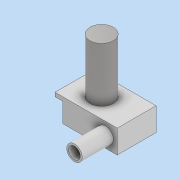
# Autodesk Inventor part: TuningPeg
Saved by Autodesk Inventor 2021 (Build 250183000, 183)
## iProperties
Created: 2021-02-02
Part Number: TuningPeg
Material: Generic
Document SubType Name: Modeling
Designer: garre
Density: 1 g/cm^3
Appearance: Default
Author: garre
Autodesk Inventor part; units mm, degrees
ref_plane "YZ Plane" through (0, 0, 0) normal (1, 0, 0) x (0, 1, 0)
ref_plane "XZ Plane" through (0, 0, 0) normal (0, 1, 0) x (-1, 0, 0)
ref_plane "XY Plane" through (0, 0, 0) normal (0, 0, 1) x (1, 0, 0)
sketch "Sketch1" plane through (0, 0, 0) normal (0, 1, 0) x (-1, 0, 0)
  circle A0 centre (0, 0) radius 4.7625
  line L0 (0, 0) -> (-14.2875, 0)
  line L1 (-14.2875, 0) -> (-14.2875, 7.9375)
  line L2 (-14.2875, 7.9375) -> (7.9375, 7.9375)
  line L3 (7.9375, 7.9375) -> (7.9375, -7.9375)
  line L4 (7.9375, -7.9375) -> (-14.2875, -7.9375)
  line L5 (-14.2875, -7.9375) -> (-14.2875, 7.9375)
  line L6 (0, -7.9375) -> (11.1125, -7.9375)
  line L7 (11.1125, -7.9375) -> (11.1125, 7.9375)
  line L8 (11.1125, 7.9375) -> (0, 7.9375)
  line L9 (0, 7.9375) -> (0, -7.9375)
  dimension "d0" = 9.525
  dimension "d9" = 15.875
  dimension "d10" = 7.9375
  dimension "d11" = 14.2875
  dimension "d12" = 7.9375
  dimension "d22" = 11.1125
  constraints: 20 end point, 4 parallel, 3 horizontal, 2 perpendicular, 1 centre point, 1 coincident, 1 midpoint, 1 point on line, 1 vertical
  measures "d0" diameter of A0
  measures "d9" distance of L4.end L1.end
  measures "d10" distance of L0.end L1.end
  measures "d11" distance from line of L5 point (0, 0)
  measures "d12" distance from line of L3 point (0, 0)
  measures "d22" distance of L6.start L6.end
extrude "Extrusion1" add sketch "Sketch1" along normal blind 31.75 contours A0 L9 | L9 L0 A0 | A0 L0 L9
extrude "Extrusion3" add sketch "Sketch1" along normal blind 9.525 separate body contours A0 L9 L2 L3 L4 | A0 L0 L1 L2 L9 | L9 L4 L5 L0 A0
sketch "Sketch3" plane through (-7.9375, 0, 7.9375) normal (0, 0, 1) x (1, 0, 0)
  line L0 (0, 0) -> (0, 9.525) projected
  line L1 (0, 4.7625) -> (22.225, 4.7625)
  line L2 (22.225, 0) -> (22.225, 9.525) projected
  circle A0 centre (17.4625, 4.7625) radius 3.175
  circle A1 centre (17.4625, 4.7625) radius 2.3813
  point P0 (7.9375, 0)
  dimension "d15" = 6.35
  dimension "d16" = 4.7625
  dimension "d17" = 4.7625
  constraints: 2 centre point, 2 end point, 2 midpoint, 1 coincident, 1 point on line
  measures "d15" diameter of A0
  measures "d16" diameter of A1
  measures "d17" distance from line of L2 A0.centre
extrude "Extrusion4" add sketch "Sketch3" along normal blind 12.7 separate body contours A1 L1 A0 | L1 A0 A1
extrude "Extrusion5" cut sketch "Sketch3" against normal up to surface (15.875 mm away) contours A1 L1 | L1 A1 bodies 2
sketch "Sketch4" plane through (0, 9.525, 0) normal (0, 1, 0) x (1, 0, 0)
  line L0 (-7.9375, -7.9375) -> (14.2875, -7.9375) projected
  line L1 (0, -7.9375) -> (-11.1125, -7.9375)
  line L2 (14.2875, 7.9375) -> (-7.9375, 7.9375) projected
  line L3 (0, 7.9375) -> (-11.1125, 7.9375)
  line L4 (-11.1125, 7.9375) -> (-11.1125, -7.9375)
  line L5 (-7.9375, 7.9375) -> (-7.9375, -7.9375) projected
  line L6 (-7.9375, -7.9375) -> (-7.9375, 7.9375)
  line L7 (0, 0) -> (0, -7.9375)
  dimension "d23" = 11.1125
  constraints: 10 end point, 2 collinear, 2 perpendicular, 2 point on line, 1 horizontal
  measures "d23" distance of L1.start L1.end
extrude "Extrusion6" add sketch "Sketch4" against normal blind 1.5875 bodies 2
equation "\"d0\" = tuningPegDiameter"
equation "\"d9\" = 2 * lockOffset"
equation "\"d10\" = lockOffset"
equation "\"d11\" = lockLongYOffset"
equation "\"d12\" = lockShortYOffset"
equation "\"d22\" = mountExtension"
equation "\"d1\" = tuningPegDepth"
equation "\"d13\" = lockWidth"
equation "\"d15\" = screwOutsideDiameter"
equation "\"d16\" = screwInsideDiameter"
equation "\"d17\" = screwOffset"
equation "\"d18\" = screwExtension"
equation "\"d20\" = screwExtension"
equation "\"d23\" = mountExtension"
equation "\"d24\" = mountPlateDepth"
equation "\"tuningPegDiameter\" = 9.525"
equation "\"tuningPegDepth\" = 31.75"
equation "\"lockWidth\" = 9.525"
equation "\"screwOffset\" = 4.7625"
equation "\"screwOutsideDiameter\" = 6.35"
equation "\"screwInsideDiameter\" = 4.7625"
equation "\"screwExtension\" = 12.7"
equation "\"mountPlateDepth\" = 1.5875"
equation "\"lockOffset\" = 7.9375"
equation "\"mountExtension\" = 11.1125"
equation "\"lockLongYOffset\" = 14.2875"
equation "\"lockShortYOffset\" = 7.9375"
body "Solid1"
body "Solid2"
body "Solid3"
